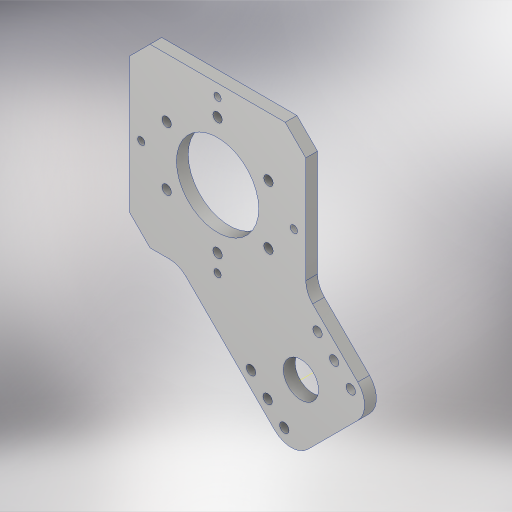
# Autodesk Inventor part: GP6-004
Saved by Autodesk Inventor 2023.4 (Build 274418000, 418)
## iProperties
RuleStatus: InUse
Created: 2025-02-23
Part Number: GP6-004
Material: Aluminum 6061
Document SubType Name: Modeling
Designer: brand
Mass: 132.735 g
Surface Area: 177.419 cm^2
Volume: 49.1612 cm^3
Density: 2.7 g/cm^3
Appearance: Aluminum - Flat
AfterDocNew0: SHOW
AfterDocOpen0: SHOW
Author: brand
Autodesk Inventor part; units mm, degrees
ref_plane "YZ Plane" through (0, 0, 0) normal (1, 0, 0) x (0, 1, 0)
ref_plane "XZ Plane" through (0, 0, 0) normal (0, 1, 0) x (-1, 0, 0)
ref_plane "XY Plane" through (0, 0, 0) normal (0, 0, 1) x (1, 0, 0)
sketch "Sketch1" plane through (0, 0, 0) normal (0, 0, 1) x (1, 0, 0)
  line L0 (-47.625, -47.625) -> (47.625, -47.625)
  line L1 (47.625, -47.625) -> (47.625, 47.625)
  line L2 (47.625, 47.625) -> (-47.625, 47.625)
  line L3 (-47.625, 47.625) -> (-47.625, -47.625)
  line L4 (-47.625, -47.625) -> (47.625, 47.625) construction
  line L5 (47.625, -47.625) -> (-47.625, 47.625) construction
  point P0 (0, 0)
  dimension "width" = 95.25
  dimension "length" = 95.25
  constraints: 12 end point, 2 midpoint, 2 parallel, 1 horizontal, 1 perpendicular
  measures "width" distance of L2.end L1.end
  measures "length" distance of L0.end L1.end
extrude "Extrusion1" add sketch "Sketch1" along normal mid plane 6.35
sketch "Sketch2" plane through (0, 0, 3.175) normal (0, 0, 1) x (1, 0, 0)
  circle A0 centre (0, 0) radius 35
  circle A1 centre (0, 0) radius 60 construction
  circle A2 centre (0, 0) radius 47.5
  line L0 (0, 35) -> (0, 60) construction
  line L1 (0, 47.5) -> (0, 35) construction
  point P0 (0, 41.25)
  point P1 (-41.25, 0)
  point P2 (0, -41.25)
  point P3 (41.25, 0)
  dimension "d4" = 70
  dimension "d5" = 120
  dimension "d8" = 360
  constraints: 4 end point, 4 vertical alignment, 3 coincident, 2 midpoint, 2 vertical, 11 other
hole "Hole1" at (0, 41.25, 3.175) at (-41.25, 0, 3.175) at (0, -41.25, 3.175) at (41.25, 0, 3.175) direction (0, 0, -1) diameter 3.9624 end through all thread size "10-32 UNF" class "2B" standard "ANSI Unified Screw Threads"
sketch "Sketch3" plane through (0, 0, 3.175) normal (0, 0, 1) x (1, 0, 0)
  circle A0 centre (0, 0) radius 31.75 construction
  point P0 (0, 31.75)
  point P1 (-27.4963, 15.875)
  point P2 (-27.4963, -15.875)
  point P3 (0, -31.75)
  point P4 (27.4963, -15.875)
  point P5 (27.4963, 15.875)
  dimension "d17" = 63.5
  dimension "d20" = 360
  constraints: 2 vertical alignment, 1 coincident, 9 other
hole "Hole2" at (0, 31.75, 3.175) at (-27.4963, 15.875, 3.175) at (-27.4963, -15.875, 3.175) at (0, -31.75, 3.175) at (27.4963, -15.875, 3.175) at (27.4963, 15.875, 3.175) direction (0, 0, -1) diameter 5.1054 end through all clearance for "Hex Machine Screw" size "#10" standard "Ansi Unified Screw Threads"
sketch "Sketch4" plane through (0, 0, 3.175) normal (0, 0, 1) x (1, 0, 0)
  circle A0 centre (0, 0) radius 22.225
  dimension "d30" = 44.45
  constraints: 1 centre point, 1 coincident
  measures "d30" diameter of A0
extrude "Extrusion2" cut sketch "Sketch4" against normal through all
sketch "Sketch5" plane through (0, 0, 3.175) normal (0, 0, 1) x (1, 0, 0)
  circle A0 centre (0, 0) radius 64 construction
  circle A1 centre (45.021, -68.5355) radius 18 construction
  line L0 (95.821, 47.9105) -> (95.821, -47.9105) construction
  line L1 (54.0013, -41.5947) -> (18.0802, -77.5157) construction
  line L2 (18.0802, -77.5157) -> (27.0605, -86.496) construction
  line L3 (36.0407, -59.5552) -> (45.021, -68.5355) construction
  line L4 (-47.625, -47.625) -> (47.625, -47.625) construction
  line L5 (-20.7907, -47.625) -> (39.7884, -108.2042)
  line L6 (39.7884, -108.2042) -> (84.6897, -63.3029)
  line L7 (84.6897, -63.3029) -> (47.625, -26.2382)
  line L8 (47.625, -47.625) -> (47.625, 47.625) construction
  line L9 (-20.7907, -47.625) -> (47.625, -47.625)
  line L10 (47.625, -47.625) -> (47.625, -26.2382)
  circle A2 centre (45.021, -68.5355) radius 9.525
  point P0 (95.821, 0)
  point P1 (27.0605, -86.496)
  point P2 (36.0407, -95.4762)
  point P3 (62.9815, -50.5749)
  point P4 (62.9815, -50.5749)
  point P5 (71.9618, -59.5552)
  point P6 (-22.225, -47.625)
  dimension "d33" = 128
  dimension "d34" = 36
  dimension "d35" = 95.821
  dimension "d36" = 95.821
  dimension "d37" = 50.8
  dimension "d38" = 12.7
  dimension "d39" = 12.7
  dimension "d42" = 12.7
  dimension "d47" = 45
  dimension "d48" = 50.8
  dimension "d49" = 6.35
  dimension "d50" = 24.35
  dimension "d51" = 6.35
  dimension "d55" = 19.05
  dimension "d64" = 45
  constraints: 18 end point, 4 coincident, 4 perpendicular, 4 symmetric about line, 3 centre point, 2 midpoint, 2 point on line, 1 collinear, 1 horizontal alignment, 1 tangent, 1 vertical, 3 other
  measures "d33" diameter of A0
  measures "d34" diameter of A1
  measures "d35" distance from line of L0 point (0, 0)
  measures "d36" distance of L0.start L0.end
  measures "d37" distance of L1.start L1.end
  measures "d38" distance of L1.end L2.end
  measures "d39" distance of L3.start L3.end
  measures "d42" distance of point (18.08, -77.516) point (27.06, -86.496)
  measures "d47" angle of L0 L3
  measures "d48" distance from line of L0 A1.centre
  measures "d49" distance from line of L7 point (54.001, -41.595)
  measures "d50" distance from line of A1.centre L6
  measures "d51" distance from line of L5 point (27.06, -86.496)
  measures "d55" diameter of A2
  measures "d64" angle of L0 L7
extrude "Extrusion3" add sketch "Sketch5" against normal up to surface (6.35 mm away)
hole "Hole3" at (18.0802, -77.5157, 3.175) at (27.0605, -86.496, 3.175) at (36.0407, -95.4762, 3.175) at (54.0013, -41.5947, 3.175) at (71.9618, -59.5552, 3.175) at (62.9815, -50.5749, 3.175) direction (0, 0, -1) diameter 5.1054 end through all clearance for "Hex Machine Screw" size "#10" standard "Ansi Unified Screw Threads"
fillet "Fillet2" radius 12.7 4 edges at (47.625, -26.2382, 0) (-20.7907, -47.625, 0) (39.7884, -108.2042, 0) (84.6897, -63.3029, 0)
sketch "Sketch7" plane through (0, 0, 3.175) normal (0, 0, 1) x (1, 0, 0)
  circle A0 centre (0, 0) radius 60 construction
  circle A1 centre (71.9618, -59.5552) radius 2.5527 construction
  circle A2 centre (36.0407, -95.4762) radius 2.5527 construction
  circle A3 centre (18.0802, -77.5157) radius 2.5527 construction
  circle A4 centre (27.0605, -86.496) radius 2.5527 construction
  circle A5 centre (54.0013, -41.5947) radius 2.5527 construction
  circle A6 centre (62.9815, -50.5749) radius 2.5527 construction
  circle A7 centre (45.021, -68.5355) radius 9.525 construction
  circle A8 centre (0, 0) radius 22.225 construction
  circle A9 centre (27.4963, -15.875) radius 2.5527 construction
  circle A10 centre (-27.4963, -15.875) radius 2.5527 construction
  circle A11 centre (0, 31.75) radius 2.5527 construction
  circle A12 centre (-27.4963, 15.875) radius 2.5527 construction
  circle A13 centre (0, -31.75) radius 2.5527 construction
  circle A14 centre (27.4963, 15.875) radius 2.5527 construction
  circle A15 centre (0, -41.25) radius 1.9812 construction
  circle A16 centre (0, 41.25) radius 1.9812 construction
  circle A17 centre (-41.25, 0) radius 1.9812 construction
  circle A18 centre (41.25, 0) radius 1.9812 construction
  arc A19 (75.7094, -72.2831) -> (75.7094, -54.3226) centre (66.7292, -63.3029) ccw construction
  line L0 (75.7094, -54.3226) -> (51.3447, -29.9579) construction
  arc A20 (47.625, -20.9777) -> (51.3447, -29.9579) centre (60.325, -20.9777) ccw construction
  line L1 (47.625, -20.9777) -> (47.625, 47.625) construction
  line L2 (47.625, 47.625) -> (-47.625, 47.625) construction
  line L3 (-47.625, 47.625) -> (-47.625, -47.625) construction
  line L4 (-47.625, -47.625) -> (-26.0513, -47.625) construction
  arc A21 (-17.071, -51.3447) -> (-26.0513, -47.625) centre (-26.0513, -60.325) ccw construction
  line L5 (-17.071, -51.3447) -> (30.8082, -99.2239) construction
  arc A22 (30.8082, -99.2239) -> (48.7687, -99.2239) centre (39.7884, -90.2436) ccw construction
  line L6 (48.7687, -99.2239) -> (75.7094, -72.2831) construction
  line L7 (-47.625, 47.625) -> (47.625, 47.625) construction
  line L8 (-36.4946, 47.625) -> (-47.625, 47.625)
  line L9 (-47.625, 47.625) -> (-47.625, 36.4946)
  line L10 (-47.625, -47.625) -> (-47.625, 47.625) construction
  line L11 (36.4946, 47.625) -> (47.625, 47.625)
  line L12 (47.625, 47.625) -> (47.625, 36.4946)
  line L13 (47.625, 47.625) -> (47.625, -20.9777) construction
  line L14 (-47.625, -36.4946) -> (-47.625, -47.625)
  line L15 (-26.0513, -47.625) -> (-47.625, -47.625) construction
  line L16 (-47.625, -47.625) -> (-36.4946, -47.625)
  line L17 (-47.625, -36.4946) -> (-36.4946, -47.625)
  line L18 (36.4946, 47.625) -> (47.625, 36.4946)
  line L19 (-36.4946, 47.625) -> (-47.625, 36.4946)
  dimension "d68" = 120
  constraints: 18 end point, 6 point on line, 3 collinear, 1 coincident, 10 other
extrude "Extrusion5" cut sketch "Sketch7" against normal through all
equation "\"d36\" = d35"
equation "\"d39\" = d38"
equation "\"d42\" = d38"
equation "\"d50\" = 0.5 * d34 + d49"
equation "\"d51\" = d49"
equation "\"d64\" = d47"
equation "\"d63\" = d29"
equation "\"d29\" = 12.7"
body "Solid1"
